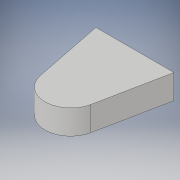
# Autodesk Inventor part: Steitenteil_voll
Saved by Autodesk Inventor 2019 (Build 230136000, 136)
## iProperties
Created: 2021-12-15
Part Number: Steitenteil_voll
Material: Generisch
Document SubType Name: Modeling
Designer: Bergi
Density: 1 g/cm^3
Appearance: Vorgabe
Author: Bergi
Autodesk Inventor part; units mm, degrees
ref_plane "YZ Plane" through (0, 0, 0) normal (1, 0, 0) x (0, 1, 0)
ref_plane "XZ Plane" through (0, 0, 0) normal (0, 1, 0) x (-1, 0, 0)
ref_plane "XY Plane" through (0, 0, 0) normal (0, 0, 1) x (1, 0, 0)
sketch "Skizze1" plane through (0, 0, 0) normal (0, 1, 0) x (-1, 0, 0)
  arc A0 (9.8057, 1.9618) -> (0, 10) centre (0, 0) ccw
  line L0 (0, -37.1505) -> (0, 19.9033) construction
  line L1 (9.8057, 1.9618) -> (16, -29)
  line L2 (16, -29) -> (0, -29)
  arc A1 (0, 10) -> (-9.8057, 1.9618) centre (0, 0) ccw
  line L3 (-9.8057, 1.9618) -> (-16, -29)
  line L4 (-16, -29) -> (0, -29)
  line L5 (15.1997, -25) -> (-15.1997, -25)
  dimension "d0" = 20
  dimension "d1" = 32
  dimension "d2" = 39
  dimension "d3" = 35
  constraints: 10 end point, 4 point on circle, 4 point on line, 2 centre point, 2 symmetric about line, 1 coincident, 1 horizontal, 1 perpendicular, 1 tangent, 1 other
  measures "d0" diameter of A0
  measures "d1" distance of L1.end L3.end
  measures "d2" distance from line of L4 A0.end
  measures "d3" distance from line of L5 A0.end
extrude "Extrusion1" add sketch "Skizze1" along normal blind 9.5 contours L1 L5 L3 A1 A0
